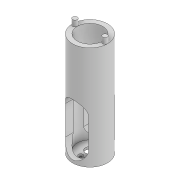
# Autodesk Inventor part: Lock
Saved by Autodesk Inventor 2020 (Build 240168000, 168)
## iProperties
Created: 2020-08-21
Part Number: Lock
Material: Generic
Document SubType Name: Modeling
Designer: Jhyatt
Density: 1 g/cm^3
Appearance: Default
Author: Jhyatt
Autodesk Inventor part; units mm, degrees
note: some values were not read from the file. Chosen so that the rebuilt part matches the saved one: direction of "Hole1".
ref_plane "YZ Plane" through (0, 0, 0) normal (1, 0, 0) x (0, 1, 0)
ref_plane "XZ Plane" through (0, 0, 0) normal (0, 1, 0) x (-1, 0, 0)
ref_plane "XY Plane" through (0, 0, 0) normal (0, 0, 1) x (1, 0, 0)
sketch "Sketch1" plane through (0, 0, 0) normal (0, 1, 0) x (-1, 0, 0)
  circle A0 centre (0, 0) radius 4
  circle A1 centre (0, 0) radius 15
  circle A2 centre (0, -8) radius 1
  circle A3 centre (0, 8) radius 1
  dimension "d0" = 30
  dimension "d1" = 8
  dimension "d2" = 8
  dimension "d3" = 2
  dimension "d4" = 2
  dimension "d5" = 8
  constraints: 4 centre point, 2 coincident
  measures "d0" diameter of A1
  measures "d1" distance of A2.centre point (0, 0)
  measures "d2" distance of point (0, 0) A3.centre
  measures "d3" diameter of A3
  measures "d4" diameter of A2
  measures "d5" diameter of A0
extrude "Extrusion1" add sketch "Sketch1" along normal blind 2
sketch "Sketch2" plane through (0, 2, 0) normal (0, 1, 0) x (1, 0, 0)
  circle A0 centre (0, 0) radius 15
  line L0 (0, 0) -> (18.7194, 0) construction
  circle A1 centre (0, 0) radius 11
  dimension "d33" = 22
  constraints: 2 centre point, 2 coincident, 2 end point, 1 horizontal
  measures "d33" diameter of A1
extrude "Extrusion2" add sketch "Sketch2" along normal blind 87
sketch "Sketch3" plane through (0, 89, 0) normal (0, 1, 0) x (1, 0, 0)
  circle A0 centre (13, 0) radius 2
  circle A1 centre (-13, 0) radius 2
  point P0 (0, 0)
  dimension "d15" = 4
  dimension "d16" = 4
  dimension "d17" = 13
  dimension "d18" = 13
  constraints: 2 centre point
  measures "d15" diameter of A0
  measures "d16" diameter of A1
  measures "d17" distance of point (0, 0) A0.centre
  measures "d18" distance of A1.centre point (0, 0)
extrude "Extrusion3" add sketch "Sketch3" along normal blind 5
sketch "Sketch4" plane through (0, 2, 0) normal (0, 1, 0) x (1, 0, 0)
  circle A0 centre (0, -8) radius 1 projected
  circle A1 centre (0, 8) radius 1 projected
  point P0 (0, 0)
  constraints: 2 coincident
hole "Hole1" at (0, 2, 8) at (0, 2, -8) direction (0, -1, 0) diameter 1.567 depth 2 countersink diameter 4 countersink angle 90 thread size "M2x0.4" class "6H" standard "ANSI Metric M Profile"
sketch "Sketch6" plane through (0, 0, 0) normal (0, 0, 1) x (1, 0, 0)
  line L0 (0, 37.5) -> (0, 12.5) construction
  line L1 (-10, 37.5) -> (-10, 12.5)
  line L2 (10, 12.5) -> (10, 37.5)
  arc A0 (10, 37.5) -> (-10, 37.5) centre (0, 37.5) ccw
  arc A1 (-10, 12.5) -> (10, 12.5) centre (0, 12.5) ccw
  line L3 (-4, 2) -> (4, 2) projected
  point P0 (0, 0)
  point P1 (0, 25)
  point P2 (-3.1225, 2)
  point P3 (3.1225, 2)
  dimension "d28" = 20
  dimension "d29" = 25
  dimension "d30" = 23
  constraints: 8 end point, 4 point on circle, 4 tangent, 2 centre point, 1 midpoint, 1 parallel, 1 vertical
  measures "d28" diameter of A1
  measures "d29" distance of L0.end L0.start
  measures "d30" distance from line of L3 point (0, 25)
extrude "Extrusion4" cut sketch "Sketch6" against normal mid plane 40
body "Solid1"
